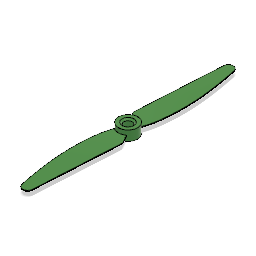
fan v1 (Autodesk Fusion 360 design; units mm, degrees)
Autodesk Fusion 360 part; units mm, degrees
sketch "Sketch1" plane through (0, 0, 0) normal (0, 1, 0) x (1, 0, 0)
  circle A0 centre (0, 0) radius 5.75
  dimension "d1" = 11.5
  constraint coincident A0.centre origin
  measures "d1" diameter of A0
extrude "Extrude1" add sketch "Sketch1" along normal mid plane 6
sketch "Sketch2" plane through (0, 0, 0) normal (0, 0, 1) x (1, 0, 0)
  line L0 (5.75, 3) -> (-5.75, 3)
  line L1 (-5.75, -3) -> (5.75, -3)
  line L2 (-5.99, 1.3829) -> (5.9749, -1.3794)
  dimension "d4" = 13
  constraint coincident origin L2
  measures "d4" angle of L1 L2
sketch "Sketch3" plane through (0, 0, 0) normal (0, 1, 0) x (1, 0, 0)
  circle A0 centre (0, 0) radius 5.75
  line L0 (-3.5598, 4.5155) -> (-6.478, 9.5938)
  line L1 (-6.478, 9.5938) -> (-3.4813, 60.953)
  spline S0 degree 5 poles (3.5598, 4.5155) (3.6773, 4.794) (3.9082, 5.3773) (4.2425, 6.332) (4.664, 7.7653) (5.1484, 9.8443) (5.5861, 12.2602) (5.9693, 15.1008) (6.2849, 18.4604) (6.5067, 22.3972) (6.6011, 26.9122) (6.5015, 31.8707) (6.167, 37.0685) (5.6191, 42.3359) (4.9052, 47.5085) (4.0907, 52.4479) (3.4107, 56.1235) (2.9079, 58.6916) (2.5788, 60.3158) (2.4158, 61.106) knots 0 0 0 0 0 0 0.066667 0.133333 0.2 0.266667 0.333333 0.4 0.466667 0.533333 0.6 0.666667 0.733333 0.8 0.866667 0.933333 1 1 1 1 1 1
  line L2 (-2.2481, 63.5) -> (-1.4613, 63.5)
  arc A1 (2.4158, 61.106) -> (-3.4633, 61.0922) centre (-0.5223, 60.5) ccw
  arc A2 (-3.4633, 61.0922) -> (-3.4813, 60.953) centre (-2.483, 60.8948) ccw
  line L3 (-3.5598, 4.5155) -> (3.5598, 4.5155) construction
  line L4 (6.5565, 20.5742) -> (6.5493, 33.2506)
  point P0 (5.1258, 9.8758)
  point P1 (6.5529, 26.9124)
  dimension "d5" = 3
  dimension "d6" = 1
  dimension "d7" = 63.5
  dimension "d9" = 12
  constraint coincident A0 L0.start
  constraint coincident A0 S0.start
  constraint horizontal L2
  constraint tangent L2 A1
  constraint tangent S0 A1
  constraint tangent L1 A2
  constraint tangent A1 A2
  constraint horizontal L3
  constraint midpoint P1 L4
  measures "d5" radius of A1
  measures "d6" radius of A2
  measures "d7" vertical distance of L2.end A0.centre
  measures "d9" distance of L1 P1
extrude "Extrude2" add sketch "Sketch3" along normal mid plane 0.6 contours A0 L0 L1 S0 A1 A2
pattern_circular "C-Pattern1" count 2 over 360 about axis through (0, 1.75, 0) along (0, 1, 0) of "Extrude2"
sketch "Sketch4" plane through (0, 3, 0) normal (0, 1, 0) x (-1, 0, 0)
  circle A0 centre (0, 0) radius 5.75
  circle A1 centre (0, 0) radius 2.5
  dimension "d16" = 5
  constraint coincident A0.centre A1.centre
  measures "d16" diameter of A1
extrude "Extrude3" cut sketch "Sketch4" against normal blind 16 contours A1
chamfer "Chamfer1" distance 1 angle 45 2 edges at (2.3308, 3, 0.904) (2.3308, -3, -0.904)
